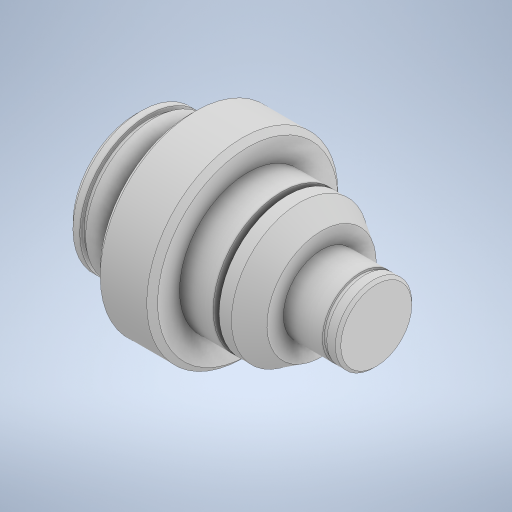
# Autodesk Inventor part: Bartosz_Zukowski_model_nr_8.ipj
Saved by Autodesk Inventor 2024 (Build 280153000, 153)
## iProperties
Created: 2024-04-11
Part Number: Bartosz_Zukowski_model_nr_8.ipj
Material: Ogólny
Document SubType Name: Modeling
Designer: Bartosz
Density: 1 g/cm^3
Appearance: Domyślna
Author: Bartosz
Autodesk Inventor part; units mm, degrees
ref_plane "YZ Plane" through (0, 0, 0) normal (1, 0, 0) x (0, 1, 0)
ref_plane "XZ Plane" through (0, 0, 0) normal (0, 1, 0) x (-1, 0, 0)
ref_plane "XY Plane" through (0, 0, 0) normal (0, 0, 1) x (1, 0, 0)
sketch "pierwsza_proba" plane through (0, 0, 0) normal (0, 0, 1) x (1, 0, 0)
  line L0 (-33.0769, 0) -> (-33.0769, 25)
  line L1 (-26.4269, 23.5) -> (-26.4269, 25)
  line L2 (-13.0769, 25) -> (-13.0769, 35)
  line L3 (-13.0769, 35) -> (7.9231, 35)
  line L4 (7.9231, 35) -> (7.9231, 25)
  line L5 (7.9231, 25) -> (20.2731, 25)
  line L6 (20.2731, 25) -> (20.2731, 22)
  line L7 (20.2731, 22) -> (22.4231, 22)
  line L8 (34.9231, 14) -> (49.2231, 14)
  line L9 (49.2231, 14) -> (49.2231, 13.3)
  line L10 (49.2231, 13.3) -> (50.8231, 13.3)
  line L11 (50.8231, 13.3) -> (50.8231, 14)
  line L12 (50.8231, 14) -> (54.9231, 14)
  line L13 (54.9231, 14) -> (54.9231, 0)
  line L14 (54.9231, 0) -> (-33.0769, 0)
  line L15 (-33.0769, 25) -> (-28.5769, 25)
  line L16 (-28.5769, 25) -> (-28.5769, 23.5)
  line L17 (-28.5769, 23.5) -> (-26.4269, 23.5)
  line L18 (-26.4269, 25) -> (-13.0769, 25)
  line L19 (22.4231, 22) -> (22.4231, 25)
  line L20 (22.4231, 25) -> (26.9231, 25)
  line L21 (34.9231, 14) -> (34.9231, 20)
  line L22 (34.9231, 20) -> (26.9231, 25)
  dimension "d6" = 88
  dimension "d7" = 5.7
  dimension "d12" = 20
  dimension "d13" = 6.65
  dimension "d14" = 70
  dimension "d15" = 50
  dimension "d16" = 47
  dimension "d18" = 28
  dimension "d19" = 26.6
  dimension "d22" = 2.15
  dimension "d23" = 2.15
  dimension "d24" = 44
  dimension "d25" = 28
  dimension "d26" = 28
  dimension "d27" = 1.6
  dimension "d28" = 50
  dimension "d42" = 34.65
  dimension "d43" = 47
  dimension "d44" = 20
  dimension "d45" = 40
  constraints: 46 end point, 12 perpendicular, 3 point on line, 2 collinear, 2 vertical, 1 horizontal
  measures "d6" distance between parallel lines of L13 L0
  measures "d7" distance between parallel lines of L13 L9
  measures "d12" distance between parallel lines of L0 L2
  measures "d13" distance between parallel lines of L0 L1
  measures "d14" diameter of L3 L14
  measures "d15" diameter of L18 L14
  measures "d16" diameter of L17 L14
  measures "d18" diameter of L12 L14
  measures "d19" diameter of L10 L14
  measures "d22" distance between parallel lines of L19 L6
  measures "d23" distance between parallel lines of L1 L16
  measures "d24" diameter of L7 L14
  measures "d25" diameter of L8 L14
  measures "d26" distance from line of L13 L20.end
  measures "d27" distance between parallel lines of L11 L9
  measures "d28" diameter of L5 L14
  measures "d42" distance between parallel lines of L13 L6
  measures "d43" distance between parallel lines of L13 L4
  measures "d44" distance from line of L13 L8.start
  measures "d45" diameter of L21.end L14
revolve "Obrót1" add sketch "pierwsza_proba" angle 360 about axis through (54.9231, 0, 0) along (-1, 0, 0)
chamfer "Faza1" distance 2 angle 45 1 edges at (-33.0769, -25, 0) measured on face at (-33.0769, 2.955, -7.7918)
chamfer "Faza2" distance 2 angle 45 1 edges at (-13.0769, -35, 0) measured on face at (-13.0769, 31.3522, 2.6905)
chamfer "Faza3" distance 2 angle 45 1 edges at (7.9231, -35, 0) measured on face at (7.9231, 31.3522, 2.6905)
chamfer "Faza4" distance 1 angle 45 1 edges at (54.9231, -14, 0) measured on face at (54.9231, -0.0766, 3.7068)
